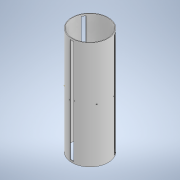
# Autodesk Inventor part: can
Saved by Autodesk Inventor 2021 (Build 250183000, 183)
## iProperties
Created: 2020-09-04
Part Number: can
Material: Generic
Document SubType Name: Modeling
Designer: dsouthall
Density: 1 g/cm^3
Appearance: Default
Author: dsouthall
Autodesk Inventor part; units mm, degrees
sketch "Sketch1" plane through (0, 0, 0) normal (0, 1, 0) x (-1, 0, 0)
  circle A0 centre (29.159538, 71.135173) radius 101.6
  circle A1 centre (29.159538, 71.135173) radius 98.425
  line L0 (29.159538, 169.560173) -> (29.159538, -27.289827) construction
  line L1 (29.159538, 71.135173) -> (41.239775, 168.816024) construction
  line L2 (29.159538, 71.135173) -> (17.0793, 168.816024) construction
  line L3 (29.159538, 71.135173) -> (97.826557, 139.802193) construction
  line L4 (29.159538, 71.135173) -> (117.147719, 121.935173) construction
  point P0 (0, 0)
  point P1 (101.001587, 142.977222)
  dimension "OD" = 203.2
  dimension "thickness" = 3.175
  dimension "d13" = 7.05
  dimension "d15" = 7.05
  dimension "end_cap_offset" = 45
  dimension "d75" = 60
  constraints: 10 end point, 6 point on circle, 2 centre point, 1 coincident, 1 point on line, 1 vertical
  measures "OD" diameter of A0
  measures "thickness" radial gap between concentric circles of A1 A0
  measures "d13" angle of L1 L0
  measures "d15" angle of L0 L2
  measures "end_cap_offset" angle of L0 L3
  measures "d75" angle of L4 L0
extrude "Extrusion1" add sketch "Sketch1" along normal blind 600
ref_plane "Work Plane1" through (-29.159538, 0, 172.735173) normal (0, 0, 1) x (1, 0, 0)
sketch "Sketch2" plane through (-29.159538, 0, 172.735173) normal (0, 0, 1) x (1, 0, 0)
  line L0 (-10, 590) -> (10, 590)
  line L1 (10, 590) -> (10, 10)
  line L2 (10, 10) -> (-10, 10)
  line L3 (-10, 10) -> (-10, 590)
  line L4 (101.6, 600) -> (-101.6, 600) projected
  line L5 (101.6, 0) -> (-101.6, 0) projected
  point P0 (29.159538, 0)
  point P1 (0, 0)
  dimension "edge_height" = 10
  dimension "d5" = 10
  dimension "slot_width" = 20
  dimension "d7" = 10
  constraints: 8 end point, 2 parallel, 1 horizontal, 1 midpoint, 1 perpendicular
  measures "edge_height" distance between parallel lines of L4 L0
  measures "d5" distance between parallel lines of L5 L2
  measures "slot_width" distance between parallel lines of L1 L3
  measures "d7" distance from line of point (0, 0) L1
extrude "Extrusion2" cut sketch "Sketch2" against normal blind 12.7
pattern_circular "Circular Pattern1" count 3 over 360 about axis through (-29.159538, 0, 71.135173) along (0, 1, 0) of "Extrusion2"
ref_plane "Central Plane" through (-29.159538, 300, 71.135173) normal (0, -1, 0) x (1, 0, 0)
ref_plane "Offset Plane A" through (-29.159538, 296.002659, 71.135173) normal (0, -1, 0) x (1, 0, 0)
ref_plane "Offset Plane B" through (-29.159538, 303.997341, 71.135173) normal (0, -1, 0) x (1, 0, 0)
ref_plane "Work Plane5" through (-41.62946, 296.002659, 171.967019) normal (-0.1227355, 0, 0.9924394) x (0, -1, 0)
ref_plane "Work Plane6" through (-16.689615, 303.997341, 171.967019) normal (0.1227355, 0, 0.9924394) x (0, 1, 0)
hole "Hole1" at (-16.689615, 303.997341, 171.967019) direction (-0.1227355, 0, -0.9924394) diameter 2.4384 depth 25.4 countersink diameter 4.699 countersink angle 82 clearance for "Flat Head Machine Screw (82)" size "#2" standard "Ansi Unified Screw Threads"
hole "Hole2" at (-41.62946, 296.002659, 171.967019) direction (0.1227355, 0, -0.9924394) diameter 2.4384 depth 25.4 tip angle 118 countersink diameter 4.699 countersink angle 82 clearance for "Flat Head Machine Screw (82)" size "#2" standard "Ansi Unified Screw Threads"
pattern_circular "Circular Pattern3" count 3 over 360 about axis through (-29.159538, 600, 71.135173) along (0, -1, 0) of "Hole1", "Hole2"
ref_plane "Work Plane7" through (-101.001587, 0, 142.977222) normal (-0.7071068, 0, 0.7071068) x (0, -1, 0)
sketch "Sketch6" plane through (-101.001587, 0, 142.977222) normal (-0.7071068, 0, 0.7071068) x (0, -1, 0)
  line L0 (0, 101.6) -> (0, -101.6) construction
  circle A0 centre (0, 0) radius 4.826 construction
  line L1 (-600, 101.6) -> (-600, -101.6) projected
  point P0 (0, -29.681257)
  point P1 (-4.826, 0)
  point P2 (-595.174, 0)
  dimension "d51" = 9.652
  dimension "d64" = 4.826
  constraints: 1 horizontal alignment, 1 midpoint, 2 other
  measures "d64" distance from line of point (-595.174, 0) L1
hole "Hole3" [suppressed]
hole "Hole4" [suppressed]
pattern_circular "Circular Pattern5" [suppressed]
ref_plane "Work Plane12" through (-117.147719, 300, 121.935173) normal (-0.8660254, 0, 0.5) x (0, -1, 0)
hole "Hole5" at (-117.147719, 300, 121.935173) direction (0.8660254, 0, -0.5) diameter 3.2766 depth 12.2936 tip angle 118 countersink diameter 5.715 countersink angle 82 clearance for "Flat Head Machine Screw (82)" size "#4" standard "Ansi Unified Screw Threads"
pattern_circular "Circular Pattern6" count 3 over 360 about axis through (-29.159538, 0, 71.135173) along (0, 1, 0) of "Hole5"
equation "\"d15\" = d13"
equation "\"d5\" = edge_height"
equation "\"d7\" = 0.5 * slot_width"
body "Solid1"
